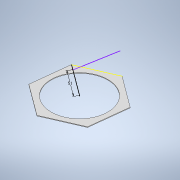
# Autodesk Inventor part: crankcase gasket
Saved by Autodesk Inventor 2020 (Build 240168000, 168)
## iProperties
Created: 2020-08-04
Part Number: crankcase gasket
Material: Generic
Document SubType Name: Modeling
Designer: benny
Density: 1 g/cm^3
Appearance: Default
Author: benny
Autodesk Inventor part; units mm, degrees
ref_plane "YZ Plane" through (0, 0, 0) normal (1, 0, 0) x (0, 1, 0)
ref_plane "XZ Plane" through (0, 0, 0) normal (0, 1, 0) x (-1, 0, 0)
ref_plane "XY Plane" through (0, 0, 0) normal (0, 0, 1) x (1, 0, 0)
sketch "Sketch3" plane through (0, 0, 0) normal (0, 1, 0) x (-1, 0, 0)
  circle A0 centre (0, 0) radius 53
  line L0 (-56.1065, -24.4416) -> (-49.2203, 36.3689)
  line L1 (-49.2203, 36.3689) -> (6.8862, 60.8105)
  line L2 (6.8862, 60.8105) -> (56.1065, 24.4416)
  line L3 (56.1065, 24.4416) -> (49.2203, -36.3689)
  line L4 (49.2203, -36.3689) -> (-6.8862, -60.8105)
  line L5 (-6.8862, -60.8105) -> (-56.1065, -24.4416)
  point P0 (-31.4964, -42.626)
  dimension "d4" = 106
  constraints: 12 end point, 2 coincident, 1 midpoint, 16 other
extrude "Extrusion2" add sketch "Sketch3" along normal blind 1
sketch "Sketch4" plane through (0, 1, 0) normal (0, 1, 0) x (1, 0, 0)
  circle A0 centre (0, 0) radius 45
  dimension "d7" = 90
  constraints: 1 centre point, 1 coincident
  measures "d7" diameter of A0
extrude "Extrusion3" cut sketch "Sketch4" against normal blind 1
sketch "Sketch5" plane through (0, 1, 0) normal (0, 1, 0) x (1, 0, 0)
  line L0 (6.8862, 60.8105) -> (-49.2203, 36.3689) projected
  line L1 (0, 0) -> (-49.2203, 36.3689)
  line L2 (0, 0) -> (-41.0175, 30.3078)
  line L3 (-41.0175, 30.3078) -> (-29.8247, 94.2463)
  dimension "d10" = 51
  constraints: 6 end point, 1 point on line
  measures "d10" distance of L1.start L2.end
body "Solid2"
